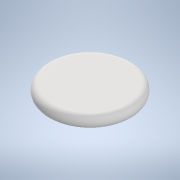
# Autodesk Inventor part: frisbee_9_000
Saved by Autodesk Inventor 2022 (Build 260153000, 153)
## iProperties
Created: 2021-04-23
Part Number: frisbee_9_000
Material: Generic
Document SubType Name: Modeling
Designer: robst
Density: 1 g/cm^3
Appearance: Default
Author: robst
Autodesk Inventor part; units mm, degrees
ref_plane "YZ Plane" through (0, 0, 0) normal (1, 0, 0) x (0, 1, 0)
ref_plane "XZ Plane" through (0, 0, 0) normal (0, 1, 0) x (-1, 0, 0)
ref_plane "XY Plane" through (0, 0, 0) normal (0, 0, 1) x (1, 0, 0)
sketch "Sketch1" plane through (0, 0, 0) normal (0, 1, 0) x (-1, 0, 0)
  circle A0 centre (0, 0) radius 114.3
  dimension "d0" = 228.6
  constraints: 1 centre point, 1 coincident
  measures "d0" diameter of A0
extrude "Extrusion1" add sketch "Sketch1" along normal mid plane 31.75
sketch "Sketch2" plane through (0, 0, 0) normal (1, 0, 0) x (0, 1, 0)
  line L0 (-15.875, 114.3) -> (-15.875, -114.3) projected
  line L1 (-15.875, -114.3) -> (15.875, -114.3) projected
  line L2 (15.875, -114.3) -> (15.875, 114.3) projected
  line L3 (-15.875, 114.3) -> (15.875, 114.3) projected
  arc A0 (-15.875, -98.425) -> (15.875, -98.425) centre (0, -98.425) ccw
  line L4 (-22.225, 0) -> (22.225, 0) projected
  point P0 (0, 0)
  point P1 (0, -114.3)
  dimension "d3" = 15.875
  constraints: 2 point on circle, 2 point on line, 1 centre point, 1 tangent
  measures "d3" distance from line of L1 A0.centre
revolve "Revolution1" cut sketch "Sketch2" angle 360 about axis through (0, -10, 0) along (0, 1, 0) contours A0 L1 L0 | A0 L2 L1
equation "\"d0\" = diameter"
equation "\"d1\" = thickness"
equation "\"diameter\" = 228.6"
equation "\"thickness\" = 31.75"
body "Solid1"
